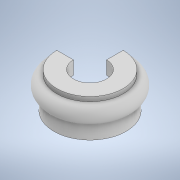
# Autodesk Inventor part: odd revolve
Saved by Autodesk Inventor 2021 (Build 250183000, 183)
## iProperties
Created: 2020-05-07
Part Number: odd revolve
Material: Generic
Document SubType Name: Modeling
Designer: david
Density: 1 g/cm^3
Appearance: Default
Author: david
Autodesk Inventor part; units mm, degrees
ref_plane "YZ Plane" through (0, 0, 0) normal (1, 0, 0) x (0, 1, 0)
ref_plane "XZ Plane" through (0, 0, 0) normal (0, 1, 0) x (-1, 0, 0)
ref_plane "XY Plane" through (0, 0, 0) normal (0, 0, 1) x (1, 0, 0)
sketch "Sketch1" plane through (0, 0, 0) normal (1, 0, 0) x (0, 1, 0)
  line L0 (21.8125, -13.0228) -> (14.2915, -13.0228)
  line L1 (14.2915, -13.0228) -> (14.2915, -22.4132)
  line L2 (14.2915, -22.4132) -> (21.8125, -22.4132)
  line L3 (21.8125, -22.4132) -> (21.8125, -13.0228)
  circle A0 centre (14.2915, -22.4132) radius 4.9585
  line L4 (11.1179, -20.5873) -> (1.6405, -20.5873)
  line L5 (1.6405, -20.5873) -> (1.6405, -24.1087)
  line L6 (1.6405, -24.1087) -> (11.1179, -24.1087)
  line L7 (11.1179, -24.1087) -> (11.1179, -20.5873)
  line L8 (21.8125, -3.6323) -> (0.6841, -3.6323)
  point P0 (0, 0)
  point P1 (14.2915, -17.4546)
  point P2 (9.6814, -20.5873)
  point P3 (9.6319, -24.1087)
  point P4 (19.25, -22.4132)
  constraints: 18 end point, 4 parallel, 3 horizontal, 2 perpendicular, 1 centre point, 1 coincident
revolve "Revolution1" add sketch "Sketch1" angle 270 about axis through (0, 21.8125, -3.6323) along (0, -1, 0)
body "Solid1"
